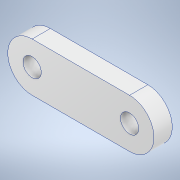
# Autodesk Inventor part: Gripper_Link
Saved by Autodesk Inventor 2021.3 (Build 253353000, 353)
## iProperties
Created: 2021-04-16
Part Number: Gripper_Link
Material: Aluminum 6061
Document SubType Name: Modeling
Designer: domin
Density: 2.7 g/cm^3
Appearance: Aluminum - Flat
Mass: 1.26464 g
Surface Area: 5.34204 cm^2
Volume: 0.468385 cm^3
Author: domin
Autodesk Inventor part; units mm, degrees
ref_plane "YZ Plane" through (0, 0, 0) normal (1, 0, 0) x (0, 1, 0)
ref_plane "XZ Plane" through (0, 0, 0) normal (0, 1, 0) x (-1, 0, 0)
ref_plane "XY Plane" through (0, 0, 0) normal (0, 0, 1) x (1, 0, 0)
sketch "Sketch1" plane through (0, 0, 0) normal (0, 0, 1) x (1, 0, 0)
  line L0 (0, 0) -> (16, 0) construction
  line L1 (0, -4) -> (16, -4)
  line L2 (16, 4) -> (0, 4)
  arc A0 (0, 4) -> (0, -4) centre (0, 0) ccw
  arc A1 (16, -4) -> (16, 4) centre (16, 0) ccw
  point P0 (8, 0)
  dimension "d0" = 16
  dimension "d1" = 8
  constraints: 8 end point, 4 point on circle, 4 tangent, 2 centre point, 1 horizontal, 1 midpoint, 1 parallel
  measures "d0" distance of L0.start L0.end
  measures "d1" diameter of A1
extrude "Extrusion1" add sketch "Sketch1" along normal blind 3
sketch "Sketch2" plane through (0, 0, 3) normal (0, 0, 1) x (1, 0, 0)
  circle A0 centre (0, 0) radius 1.5
  arc A1 (16, -4) -> (16, 4) centre (16, 0) ccw projected
  circle A2 centre (16, 0) radius 1.5
  dimension "d4" = 3
  dimension "d5" = 3
  constraints: 2 centre point, 2 coincident
  measures "d4" diameter of A0
  measures "d5" diameter of A2
hole "Hole1" at (0, 0, 3) at (16, 0, 3) direction (0, 0, -1) diameter 3 end through all
equation "\"d6\" = d4"
body "Solid1"
